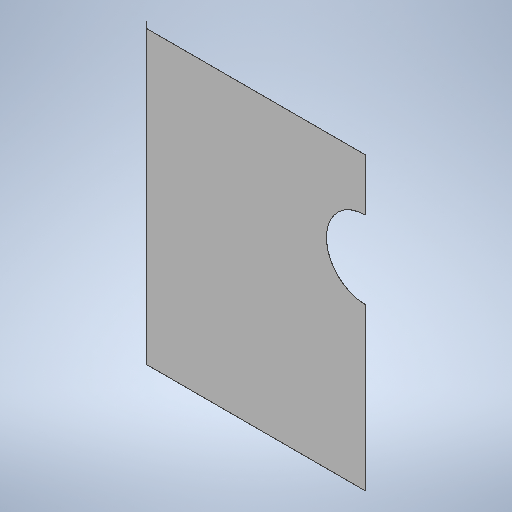
# Autodesk Inventor part: GBK-RK-0018 long wall 4
Saved by Autodesk Inventor 2026 (Build 300175000, 175)
## iProperties
Created: 2026-09-14
Part Number: GBK-RK-0018 long wall 4
Material: Generic
Document SubType Name: Sheet Metal
Designer: admin
Density: 1 g/cm^3
Sheet Metal Rule: По умолчанию_мм
Appearance: Default
Author: admin
Autodesk Inventor part; units mm, degrees
ref_plane "YZ Plane" through (0, 0, 0) normal (1, 0, 0) x (0, 1, 0)
ref_plane "XZ Plane" through (0, 0, 0) normal (0, 1, 0) x (-1, 0, 0)
ref_plane "XY Plane" through (0, 0, 0) normal (0, 0, 1) x (1, 0, 0)
sketch "Sketch1" plane through (0, 0, 0) normal (1, 0, 0) x (0, 1, 0)
  line L0 (1620, 0) -> (70, 0)
  line L1 (70, 0) -> (20, 0)
  line L2 (20, 0) -> (0, 0)
  dimension "d0" = 180
  dimension "d1" = 50
  dimension "d2" = 1620
  dimension "d3" = 20
  measures "d0" angle of L1 L0
  measures "d1" distance of L0.end L1.end
  measures "d2" distance of L0.start L2.end
  measures "d3" distance of L1.end L2.end
contour flange "Contour Flange1" sketch "Sketch1" thickness 0.5 bend radius 0.5 width 1200 along (-1, 0, 0) mid plane no both sides no wall seen from (0, 845, 0) lies toward (0, 0, 1) curves L0 L1
bend "Bend1"
corner "Corner1"
sketch "Sketch2" plane through (-1199.6464, 1620, 0.1464) normal (-0.7071068, 0, 0.7071068) x (0, -1, 0)
  line L0 (1600, 0) -> (0, 0)
  line L1 (0, 0) -> (0, -50)
  line L2 (0, -50) -> (1600, -50)
  line L3 (1600, -50) -> (1600, 0)
  constraints: 6 end point, 1 horizontal, 1 perpendicular, 1 vertical
edge flange "Flange1" height 50 angle 45 thickness 0.5 bend radius 0.5 thickness toward (-0.7071068, 0, 0.7071068) relief straight relief width 0.5 relief depth 0.25 corner gap 0.5 corner form 0 edges at (-1200, 845, 0) (-1200, 45, 0) wall of the first edge with corners at (-1199.6464, 20, 0.1464) (-1199.6464, 1620, 0.1464) (-1235.0018, 1620, -35.2089) (-1235.0018, 20, -35.2089)
bend "Bend2"
corner "Corner2"
sketch "Sketch3" plane through (0, 49.7046, 0) normal (0, 0, -1) x (1, 0, 0)
  line L0 (-1199.5858, 29.7046) -> (-1199.5858, -1570.2954) construction
  line L1 (0, 29.7046) -> (0, -1570.2954) projected
  line L2 (0, -1570.2954) -> (-1199.5858, -1570.2954) construction
  line L3 (0, -1570.2954) -> (0, 29.7046) projected
  circle A0 centre (0, -1070.2954) radius 213
  line L4 (-1199.5858, 29.7046) -> (0, 29.7046) projected
  point P0 (0, 49.7046)
  point P1 (0, 0)
  point P2 (0, -1283.2954)
  point P3 (0, -857.2954)
  dimension "d25" = 426
  dimension "d29" = 500
  constraints: 2 end point, 1 centre point, 1 point on line
  measures "d25" diameter of A0
  measures "d29" distance from line of L2 A0.centre
extrude "Cut1" cut sketch "Sketch3" against normal blind 0.5
equation "\"d27\" = Thickness"
equation "\"d4\" = Thickness"
equation "\"d5\" = BendReliefWidth"
equation "\"d6\" = BendReliefDepth"
equation "\"d7\" = MinimumRemnant"
equation "\"d8\" = TransitionRadius"
equation "\"d10\" = BendRadius"
equation "\"d12\" = CornerReliefSize"
equation "\"d13\" = GapSize"
equation "\"d14\" = JacobiRadiusSize"
equation "\"d15\" = BendReliefWidth"
equation "\"d16\" = BendReliefDepth"
equation "\"d17\" = MinimumRemnant"
equation "\"d18\" = TransitionRadius"
equation "\"d21\" = BendRadius"
equation "\"d22\" = CornerReliefSize"
equation "\"d23\" = GapSize"
equation "\"d24\" = JacobiRadiusSize"
equation "\"BendRadius\" = Thickness"
equation "\"BendReliefWidth\" = Thickness"
equation "\"BendReliefDepth\" = 0.5 * Thickness"
equation "\"CornerReliefSize\" = 4 * Thickness"
equation "\"MinimumRemnant\" = 2 * Thickness"
equation "\"TransitionRadius\" = BendRadius"
equation "\"JacobiRadiusSize\" = BendRadius"
equation "\"GapSize\" = Thickness"
equation "\"Thickness\" = 0.5"
body "Solid1"
